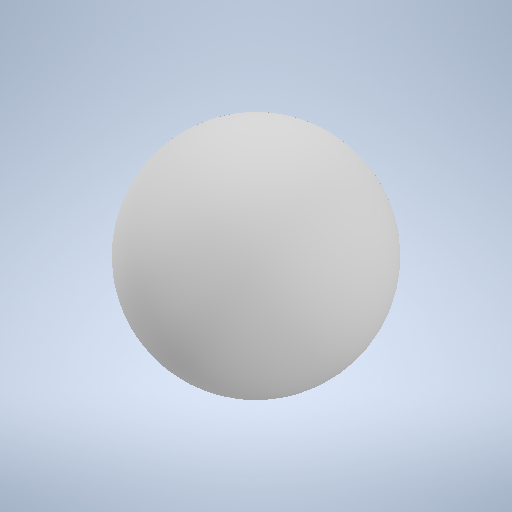
# Autodesk Inventor part: Peça1_esfera
Saved by Autodesk Inventor 2025.2 (Build 292293000, 293)
## iProperties
Created: 2025-03-26
Part Number: Peça1_esfera
Material: Genérico
Document SubType Name: Modeling
Designer: Formação
Density: 1 g/cm^3
Appearance: Padrão
Author: Formação
Autodesk Inventor part; units mm, degrees
ref_plane "YZ Plane" through (0, 0, 0) normal (1, 0, 0) x (0, 1, 0)
ref_plane "XZ Plane" through (0, 0, 0) normal (0, 1, 0) x (-1, 0, 0)
ref_plane "XY Plane" through (0, 0, 0) normal (0, 0, 1) x (1, 0, 0)
sketch "Esboço3" plane through (0, 0, 0) normal (0, 0, 1) x (1, 0, 0)
  line L0 (-10, 0) -> (10, 0) construction
  arc A0 (0, -10) -> (0, 10) centre (0, 0) ccw
  line L1 (0, 10) -> (0, -10)
  line L2 (-14, 0) -> (14, 0) projected
  line L3 (0, -14) -> (0, 14) projected
  dimension "d16" = 20
  constraints: 6 coincident, 4 end point, 3 point on circle, 2 midpoint, 1 centre point, 1 horizontal, 1 vertical
  measures "d16" distance of L1.end L1.start
revolve "Revolução1" add sketch "Esboço3" angle 360 mid plane about axis through (0, -10, 0) along (0, 1, 0)
